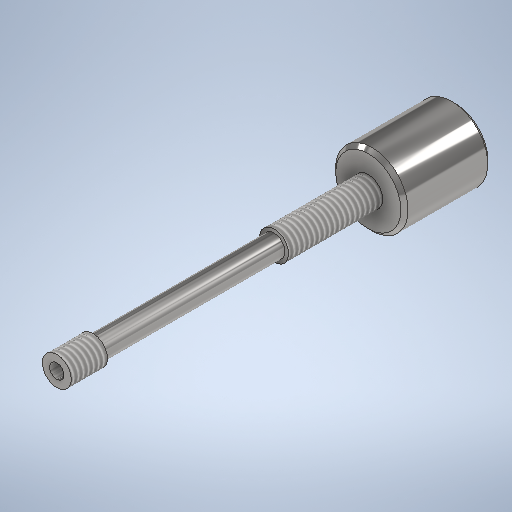
# Autodesk Inventor part: HeatBreak_HotEnd
Saved by Autodesk Inventor 2025.2 (Build 292293000, 293)
## iProperties
Created: 2026-06-11
Part Number: HeatBreak_HotEnd
Material: Generic
Document SubType Name: Modeling
Designer: Simon
Density: 1 g/cm^3
Appearance: Steel - Polished
Author: Simon
Autodesk Inventor part; units mm, degrees
ref_plane "YZ Plane" through (0, 0, 0) normal (1, 0, 0) x (0, 1, 0)
ref_plane "XZ Plane" through (0, 0, 0) normal (0, 1, 0) x (-1, 0, 0)
ref_plane "XY Plane" through (0, 0, 0) normal (0, 0, 1) x (1, 0, 0)
sketch "Sketch1" plane through (0, 0, 0) normal (1, 0, 0) x (0, 1, 0)
  line L0 (0, 0) -> (1, 0)
  line L1 (1, 0) -> (1, -55)
  line L2 (1, -55) -> (0, -55)
  line L3 (0, -55) -> (0, 0)
  line L4 (0, -55) -> (3, -55)
  line L5 (3, -55) -> (3, -50)
  line L6 (0, -55) -> (5, -55)
  line L7 (5, -55) -> (5, -50)
  line L8 (5, -50) -> (0, -50)
  line L9 (5, -50) -> (5, -43)
  line L10 (5, -43) -> (0, -43)
  line L11 (0, -43) -> (2, -43)
  line L12 (2, -43) -> (2, -30)
  line L13 (2, -30) -> (0, -30)
  line L14 (0, -30) -> (1.5, -30)
  line L15 (1.5, -30) -> (1.5, -5)
  line L16 (1.5, -5) -> (0, -5)
  line L17 (0, -5) -> (2, -5)
  line L18 (2, -5) -> (2, 0)
  line L19 (2, 0) -> (0, 0)
  line L20 (5, -43) -> (5, -44.5)
  line L21 (5, -44.5) -> (0, -44.5)
  line L22 (0, -50) -> (2.5, -50)
  line L23 (2.5, -50) -> (2.5, -44.5)
  point P0 (1, -50)
  point P1 (1, -44.5)
  dimension "d0" = 1
  dimension "d1" = 55
  dimension "d2" = 3
  dimension "d3" = 5
  dimension "d4" = 5
  dimension "d5" = 7
  dimension "d6" = 2
  dimension "d7" = 13
  dimension "d8" = 1.5
  dimension "d9" = 25
  dimension "d10" = 5
  dimension "d22" = 5
  dimension "d23" = 1.5
  constraints: 48 end point, 14 perpendicular, 10 point on line, 3 horizontal, 2 midpoint, 1 vertical
  measures "d0" distance of L0.start L0.end
  measures "d1" distance of L0.end L1.end
  measures "d2" distance of L2.end L4.end
  measures "d3" distance of L4.end L5.end
  measures "d4" distance of L2.end L6.end
  measures "d5" distance of L7.end L9.end
  measures "d6" distance of L10.end L11.end
  measures "d7" distance of L11.end L12.end
  measures "d8" distance of L13.end L14.end
  measures "d9" distance of L14.end L15.end
  measures "d10" distance of L17.end L18.end
  measures "d22" distance of L6.end L7.end
  measures "d23" distance of L9.end L20.end
revolve "Revolution1" add sketch "Sketch1" angle 360 about axis through (0, 0, -55) along (0, 0, 1) contours L19 L18 L17 L16 L1 | L16 L15 L13 L1 | L13 L12 L10 L1 | L10 L9 L21 L1 | L21 L9 L8 L23 | L5 L8 L7 L6
thread "Thread1" size "M4x0.7" class "6g" standard "ISO Metric profile" full length
thread "Thread2" size "M4x0.7" class "6g" standard "ANSI Metric M Profile" full length
thread "Thread3" size "M6x1" class "6H" standard "ANSI Metric M Profile" full length
chamfer "Chamfer1" distance 0.5 angle 45 3 edges at (0, -5, -55) (0, -5, -43) (0, -3, -55)
body "Solid1"
